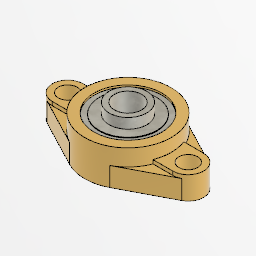
fusion (Autodesk Fusion 360 design; units mm, degrees)
Autodesk Fusion 360 part; units mm, degrees
sketch "Sketch1" plane through (0, 0, 0) normal (0, 0, 1) x (1, 0, 0)
  circle A0 centre (0, 0) radius 115
  circle A1 centre (-160, 0) radius 41
  line L0 (-178.9625, 36.3514) -> (-53.1875, 101.9612)
  line L1 (-178.9625, -36.3514) -> (-53.1875, -101.9612)
  line L2 (0, 2.5) -> (0, 20)
  line L3 (178.9625, 36.3514) -> (53.1875, 101.9612)
  circle A2 centre (160, 0) radius 41
  line L4 (178.9625, -36.3514) -> (53.1875, -101.9612)
  dimension "d1" = 115
  dimension "d3" = 41
  dimension "d4" = 160
  measures "d1" radius of A0
  measures "d3" radius of A1
  measures "d4" distance of A0.centre A1.centre
extrude "Extrude1" add sketch "Sketch1" along normal blind 51 makes body 1
sketch "Sketch2" plane through (0, 0, 51) normal (0, 0, 1) x (-1, 0, 0)
  line L0 (-178.9625, -36.3514) -> (-53.1875, -101.9612)
  arc A0 (-53.1875, -101.9612) -> (53.1875, -101.9612) centre (0, 0) ccw
  line L1 (53.1875, -101.9612) -> (178.9625, -36.3514)
  arc A1 (178.9625, -36.3514) -> (178.9625, 36.3514) centre (160, 0) ccw
  line L2 (178.9625, 36.3514) -> (53.1875, 101.9612)
  arc A2 (53.1875, 101.9612) -> (-53.1875, 101.9612) centre (0, 0) ccw
  line L3 (-53.1875, 101.9612) -> (-178.9625, 36.3514)
  arc A3 (-178.9625, 36.3514) -> (-178.9625, -36.3514) centre (-160, 0) ccw
  circle A4 centre (160, 0) radius 25
  circle A5 centre (160, 0) radius 41
  circle A6 centre (0, 0) radius 115
  line L4 (160, 41) -> (107.443, 41)
  line L5 (160, -41) -> (107.443, -41)
  line L6 (0, -2.5) -> (0, -20) construction
  line L7 (-160, -41) -> (-107.443, -41)
  circle A7 centre (-160, 0) radius 25
  line L8 (-160, 41) -> (-107.443, 41)
  circle A8 centre (-160, 0) radius 41
  dimension "d7" = 25
  measures "d7" radius of A4
extrude "Extrude2" add sketch "Sketch2" along normal blind 10 contours A3 A8 | A6 L7 L8 A8 | A1 A5 | A5 A6 L4 L5 bodies 1
sketch "Sketch3" plane through (0, 0, 51) normal (0, 0, 1) x (-1, 0, 0)
  arc A0 (178.9625, 36.3514) -> (160, 41) centre (160, 0) ccw
  line L0 (178.9625, 36.3514) -> (53.1875, 101.9612)
  arc A1 (53.1875, 101.9612) -> (-53.1875, 101.9612) centre (0, 0) ccw
  line L1 (-53.1875, 101.9612) -> (-178.9625, 36.3514)
  arc A2 (-160, 41) -> (-178.9625, 36.3514) centre (-160, 0) ccw
  line L2 (-160, 41) -> (-107.443, 41)
  arc A3 (-107.443, 41) -> (-107.443, -41) centre (0, 0) ccw
  line L3 (-107.443, -41) -> (-160, -41)
  arc A4 (-178.9625, -36.3514) -> (-160, -41) centre (-160, 0) ccw
  line L4 (-178.9625, -36.3514) -> (-53.1875, -101.9612)
  arc A5 (-53.1875, -101.9612) -> (53.1875, -101.9612) centre (0, 0) ccw
  line L5 (53.1875, -101.9612) -> (178.9625, -36.3514)
  arc A6 (160, -41) -> (178.9625, -36.3514) centre (160, 0) ccw
  line L6 (160, -41) -> (107.443, -41)
  arc A7 (107.443, -41) -> (107.443, 41) centre (0, 0) ccw
  line L7 (107.443, 41) -> (160, 41)
  circle A8 centre (0, 0) radius 90
  circle A9 centre (0, 0) radius 115
  dimension "d10" = 90
  measures "d10" radius of A8
extrude "Extrude3" add sketch "Sketch3" along normal blind 44 contours A1 A3 A5 A7 A9 bodies 1
extrude "Extrude4" cut 3 faces at (-154.8043, 1.6027, 51) (15, -25.9808, 51) (165.1957, 1.6027, 51) along direction (0, 0, -1) through all on bodies 1 bodies 1
sketch "Sketch4" plane through (0, 0, 0) normal (0, 0, 1) x (1, 0, 0)
  circle A0 centre (0, 0) radius 76
  circle A1 centre (0, 0) radius 50
  circle A2 centre (0, 0) radius 36
  circle A3 centre (0, 0) radius 90
  dimension "d14" = 76
  dimension "d15" = 50
  dimension "d16" = 36
  measures "d14" radius of A0
  measures "d15" radius of A1
  measures "d16" radius of A2
extrude "Extrude5" add sketch "Sketch4" along normal blind 90 separate body contours A3 makes body 2
extrude "Extrude6" add sketch "Sketch4" along normal blind 92 separate body contours A0 makes body 3
extrude "Extrude7" add sketch "Sketch4" along normal blind 119 separate body contours A1 makes body 4
equation "d4 = ( 320 / 2 ) * 1 mm"
equation "d21 = 51 mm + 44 mm + 24 mm"
